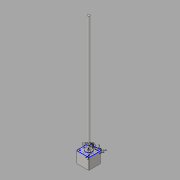
# Autodesk Inventor part: nema17
Saved by Autodesk Inventor 2016 (Build 200138000, 138)
## iProperties
Created: 2015-10-11
Part Number: nema17
Material: Generic
Document SubType Name: Modeling
Designer: daniel
Density: 1 g/cm^3
Appearance: Default
Author: daniel
Autodesk Inventor part; units mm, degrees
ref_plane "YZ Plane" through (0, 0, 0) normal (1, 0, 0) x (0, 1, 0)
ref_plane "XZ Plane" through (0, 0, 0) normal (0, 1, 0) x (-1, 0, 0)
ref_plane "XY Plane" through (0, 0, 0) normal (0, 0, 1) x (1, 0, 0)
sketch "Sketch1" plane through (0, 0, 0) normal (0, 0, 1) x (1, 0, 0)
  line L0 (-19.15, 21.15) -> (19.15, 21.15)
  line L1 (19.15, 21.15) -> (21.15, 19.15)
  line L2 (21.15, 19.15) -> (21.15, -19.15)
  line L3 (21.15, -19.15) -> (19.15, -21.15)
  line L4 (19.15, -21.15) -> (-19.15, -21.15)
  line L5 (-19.15, -21.15) -> (-21.15, -19.15)
  line L6 (-21.15, -19.15) -> (-21.15, 19.15)
  line L7 (-21.15, 19.15) -> (-19.15, 21.15)
  circle A0 centre (-15.5, 15.5) radius 1.5
  circle A1 centre (15.5, 15.5) radius 1.5
  circle A2 centre (15.5, -15.5) radius 1.5
  circle A3 centre (-15.5, -15.5) radius 1.5
  line L8 (-15.5, 15.5) -> (-15.5, -15.5) construction
  line L9 (15.5, 15.5) -> (-15.5, 15.5) construction
  line L10 (-15.5, -15.5) -> (15.5, -15.5) construction
  line L11 (15.5, 15.5) -> (15.5, -15.5) construction
  line L12 (0, 21.15) -> (0, -21.15) construction
  line L13 (-21.15, 0) -> (21.15, 0) construction
  circle A4 centre (0, 0) radius 11
  point P0 (0, 0)
  point P1 (0, 15.5)
  point P2 (-15.5, 0)
  dimension "d0" = 135
  dimension "d1" = 42.3
  dimension "d2" = 2
  dimension "d4" = 31
  dimension "d6" = 3
  dimension "d7" = 22
  constraints: 30 end point, 7 midpoint, 6 coincident, 6 parallel, 5 centre point, 5 equal length, 4 point on line, 3 equal radius, 3 perpendicular, 2 vertical, 1 horizontal
  measures "d0" angle of L7 L6
  measures "d1" distance between parallel lines of L2 L6
  measures "d2" horizontal distance of L1.end L0.end
  measures "d4" distance between parallel lines of L11 L8
  measures "d6" diameter of A2
  measures "d7" diameter of A4
extrude "Extrusion1" add sketch "Sketch1" along normal blind 2 contours A4
extrude "Extrusion2" add sketch "Sketch1" against normal blind 39 contours L0 L1 L2 L3 L4 L5 L6 L7 | A4
sketch "Sketch2" plane through (0, 0, 2) normal (0, 0, 1) x (1, 0, 0)
  circle A0 centre (0, 0) radius 4
  dimension "d12" = 8
  constraints: 1 centre point, 1 coincident
  measures "d12" diameter of A0
extrude "Extrusion3" add sketch "Sketch2" along normal blind 400
body "Solid1"
